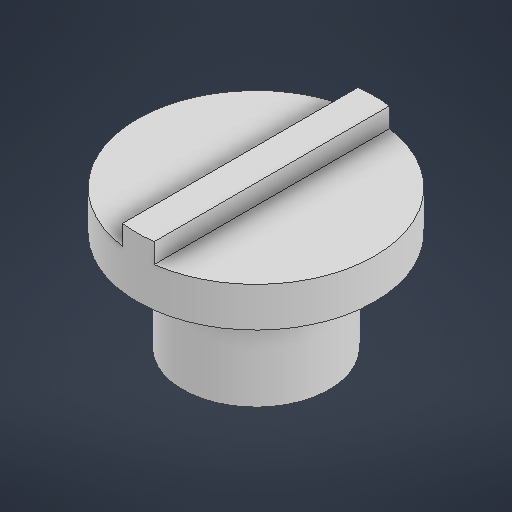
# Autodesk Inventor part: PrzegubGorny
Saved by Autodesk Inventor 2026 (Build 300175000, 175)
## iProperties
Created: 2025-05-01
Part Number: PrzegubGorny
Material: Generic
Document SubType Name: Modeling
Designer: isan
Density: 1 g/cm^3
Appearance: Default
Author: isan
Autodesk Inventor part; units mm, degrees
ref_plane "YZ Plane" through (0, 0, 0) normal (1, 0, 0) x (0, 1, 0)
ref_plane "XZ Plane" through (0, 0, 0) normal (0, 1, 0) x (-1, 0, 0)
ref_plane "XY Plane" through (0, 0, 0) normal (0, 0, 1) x (1, 0, 0)
sketch "Sketch1" plane through (0, 0, 0) normal (0, 0, 1) x (1, 0, 0)
  circle A0 centre (0, 0) radius 6
  dimension "d0" = 12
  constraints: 1 centre point, 1 coincident
  measures "d0" diameter of A0
extrude "Extrusion1" add sketch "Sketch1" along normal blind 2
sketch "Sketch2" plane through (0, 0, 2) normal (0, 0, 1) x (1, 0, 0)
  line L0 (-0.8, -7.5) -> (0.8, -7.5)
  line L1 (0.8, -7.5) -> (0.8, 7.5)
  line L2 (0.8, 7.5) -> (-0.8, 7.5)
  line L3 (-0.8, 7.5) -> (-0.8, -7.5)
  line L4 (-0.8, -7.5) -> (0.8, 7.5) construction
  line L5 (0.8, -7.5) -> (-0.8, 7.5) construction
  circle A0 centre (0, 0) radius 6 projected
  line L6 (-6, 0) -> (6, 0) construction
  point P0 (0.8, 5.9464)
  point P1 (-0.8, 5.9464)
  point P2 (-0.8, -5.9464)
  point P3 (0.8, -5.9464)
  dimension "d5" = 1.6
  dimension "d6" = 15
  constraints: 14 end point, 4 midpoint, 2 horizontal, 2 parallel, 2 point on circle, 1 perpendicular
  measures "d5" distance of L1.end L2.end
  measures "d6" distance of L0.end L1.end
extrude "Extrusion2" add sketch "Sketch2" along normal blind 1 contours L3 A0 L1
sketch "Sketch3" plane through (0, 0, 0) normal (0, 0, -1) x (-1, 0, 0)
  circle A0 centre (0, 0) radius 3.7
  dimension "d9" = 7.4
  constraints: 1 centre point, 1 coincident
  measures "d9" diameter of A0
extrude "Extrusion3" add sketch "Sketch3" along normal blind 5
sketch "Sketch4" plane through (0, 0, -5) normal (0, 0, -1) x (-1, 0, 0)
  circle A0 centre (0, 0) radius 1.7
  dimension "d12" = 3.4
  constraints: 1 centre point, 1 coincident
  measures "d12" diameter of A0
extrude "Extrusion4" cut sketch "Sketch4" against normal blind 5
body "Solid1"
